# Autodesk Inventor part: MOSFET-NCHANNEL2N7002PW
Saved by Autodesk Inventor 2016 SP1 (Build 200210100, 210)
## iProperties
Created: 2015-11-19
Part Number: MOSFET-NCHANNEL2N7002PW
Material: Generic
Document SubType Name: Modeling
Designer: PhillipD
Density: 1 g/cm^3
Appearance: SOT323, MOSFET-NCHANNEL2N7002PW
Author: PhillipD
Autodesk Inventor part; units mm, degrees
ref_plane "YZ Plane" through (0, 0, 0) normal (1, 0, 0) x (0, 1, 0)
ref_plane "XZ Plane" through (0, 0, 0) normal (0, 1, 0) x (-1, 0, 0)
ref_plane "XY Plane" through (0, 0, 0) normal (0, 0, 1) x (1, 0, 0)
sketch "SOT323, MOSFET-NCHANNEL2N7002PW_32" plane through (0, 0, 0) normal (0, 0, 1) x (1, 0, 0)
  line L0 (-1.1224, 0.7366) -> (1.1986, 0.7366)
  line L1 (1.1986, 0.7366) -> (1.1986, -0.7366)
  line L2 (1.1986, -0.7366) -> (-1.1224, -0.7366)
  line L3 (-1.1224, -0.7366) -> (-1.1224, 0.7366)
  constraints: 8 end point
extrude "Extrusion1" add sketch "SOT323, MOSFET-NCHANNEL2N7002PW_32" along normal blind 1
body "Solid1"
